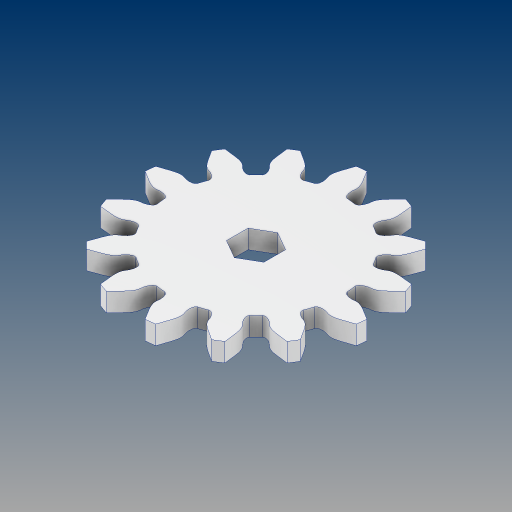
# Autodesk Inventor part: SHOT_1_016_5DP14TGear
Saved by Autodesk Inventor 2024.3 (Build 283343000, 343)
## iProperties
Created: 2024-08-09
Part Number: SHOT_1_016_5DP14TGear
Material: Aluminum 6061
Document SubType Name: Modeling
Designer: Kenji
Density: 2.7 g/cm^3
Appearance: Aluminum - Flat
Author: Kenji
Autodesk Inventor part; units mm, degrees
ref_plane "YZ Plane" through (0, 0, 0) normal (1, 0, 0) x (0, 1, 0)
ref_plane "XZ Plane" through (0, 0, 0) normal (0, 1, 0) x (-1, 0, 0)
ref_plane "XY Plane" through (0, 0, 0) normal (0, 0, 1) x (1, 0, 0)
sketch "Sketch3" plane through (0, 0, 0) normal (0, 1, 0) x (-1, 0, 0)
  circle A0 centre (0, 0) radius 40.64
  circle A1 centre (0, 0) radius 35.56 construction
  line L0 (0, 0) -> (0, -35.56) construction
  line L1 (0, 0) -> (11.4288, -31.4003) construction
  line L2 (11.4288, -31.4003) -> (0, -35.56) construction
  arc A2 (11.4288, -31.4003) -> (20.9412, -26.0395) centre (0, 0) ccw construction
  arc A3 (-0.498, -33.4118) -> (11.4288, -31.4003) centre (0, 0) ccw construction
  line L3 (20.9412, -26.0395) -> (2.9165, -40.5352) construction
  line L4 (0, -35.56) -> (-0.498, -33.4118) construction
  line L5 (26.4425, -30.8611) -> (-29.9661, -27.4526) construction
  line L6 (-0.498, -33.4118) -> (-1.7618, -29.1568) construction
  line L7 (15.9914, -37.3615) -> (-36.81, -17.2231) construction
  line L8 (-0.498, -33.4118) -> (-0.4624, -31.086) construction
  line L9 (-0.4624, -31.086) -> (-1.7618, -29.1568) construction
  line L10 (12.7503, -38.5881) -> (-38.1434, -14.0245) construction
  line L11 (-0.498, -33.4118) -> (-0.3808, -32.2504) construction
  line L12 (-0.3808, -32.2504) -> (-0.4624, -31.086) construction
  line L13 (20.121, -35.3094) -> (-34.6219, -21.2823) construction
  line L14 (-0.498, -33.4118) -> (-0.8403, -29.9384) construction
  line L15 (-0.8403, -29.9384) -> (-1.7618, -29.1568) construction
  line L16 (-0.4624, -31.086) -> (-0.8403, -29.9384) construction
  line L17 (0, 0) -> (-3.2705, -29.0263) construction
  circle A4 centre (0, 0) radius 29.21 construction
  spline S0 degree 4 poles (2.9165, -40.5352) (1.7773, -38.368) (-1.3084, -34.6409) (0.0656, -32.8612) (-0.5512, -30.4753) (-0.8986, -29.4269) (-1.7618, -29.1568) knots 0 0 0 0 0 0.524578 0.668441 1 1 1 1 1
  arc A5 (-3.2705, -29.0263) -> (-1.7618, -29.1568) centre (0, 0) ccw
  spline S1 degree 4 poles (-11.8633, -38.8699) (-10.2705, -37.0106) (-6.4328, -34.0635) (-7.3763, -32.0227) (-6.244, -29.8339) (-5.672, -28.889) (-4.7704, -28.8178) knots 0 0 0 0 0 0.524578 0.668441 1 1 1 1 1
  arc A6 (-4.7704, -28.8178) -> (-3.2705, -29.0263) centre (0, 0) ccw
  arc A7 (9.6475, -27.5708) -> (11.0634, -27.0338) centre (0, 0) ccw
  arc A8 (8.2056, -28.0338) -> (9.6475, -27.5708) centre (0, 0) ccw
  spline S2 degree 4 poles (6.1766, -40.1679) (6.8049, -37.8016) (8.9839, -33.4812) (7.2483, -32.0519) (7.3188, -29.5886) (7.4242, -28.4891) (8.2056, -28.0338) knots 0 0 0 0 0 0.524578 0.668441 1 1 1 1 1
  spline S3 degree 4 poles (20.2152, -35.2555) (18.2486, -33.7973) (13.8513, -31.778) (14.3171, -29.5785) (12.7261, -27.6965) (11.9582, -26.9026) (11.0634, -27.0338) knots 0 0 0 0 0 0.524578 0.668441 1 1 1 1 1
  arc A9 (20.6546, -20.6546) -> (21.6973, -19.5564) centre (0, 0) ccw
  arc A10 (19.5564, -21.6973) -> (20.6546, -20.6546) centre (0, 0) ccw
  spline S4 degree 4 poles (22.9931, -33.5101) (22.5325, -31.1055) (22.6211, -26.2676) (20.4373, -25.7329) (19.432, -23.4829) (19.0499, -22.4466) (19.5564, -21.6973) knots 0 0 0 0 0 0.524578 0.668441 1 1 1 1 1
  spline S5 degree 4 poles (33.5101, -22.9931) (31.1055, -22.5325) (26.2676, -22.6211) (25.7329, -20.4373) (23.4829, -19.432) (22.4466, -19.0499) (21.6973, -19.5564) knots 0 0 0 0 0 0.524578 0.668441 1 1 1 1 1
  arc A11 (27.5708, -9.6475) -> (28.0338, -8.2056) centre (0, 0) ccw
  arc A12 (27.0338, -11.0634) -> (27.5708, -9.6475) centre (0, 0) ccw
  spline S6 degree 4 poles (35.2555, -20.2152) (33.7973, -18.2486) (31.778, -13.8513) (29.5785, -14.3171) (27.6965, -12.7261) (26.9026, -11.9582) (27.0338, -11.0634) knots 0 0 0 0 0 0.524578 0.668441 1 1 1 1 1
  spline S7 degree 4 poles (40.1679, -6.1766) (37.8016, -6.8049) (33.4812, -8.9839) (32.0519, -7.2483) (29.5886, -7.3188) (28.4891, -7.4242) (28.0338, -8.2056) knots 0 0 0 0 0 0.524578 0.668441 1 1 1 1 1
  arc A13 (29.0263, 3.2705) -> (28.8178, 4.7704) centre (0, 0) ccw
  arc A14 (29.1568, 1.7618) -> (29.0263, 3.2705) centre (0, 0) ccw
  spline S8 degree 4 poles (40.5352, -2.9165) (38.368, -1.7773) (34.6409, 1.3084) (32.8612, -0.0656) (30.4753, 0.5512) (29.4269, 0.8986) (29.1568, 1.7618) knots 0 0 0 0 0 0.524578 0.668441 1 1 1 1 1
  spline S9 degree 4 poles (38.8699, 11.8633) (37.0106, 10.2705) (34.0635, 6.4328) (32.0227, 7.3763) (29.8339, 6.244) (28.889, 5.672) (28.8178, 4.7704) knots 0 0 0 0 0 0.524578 0.668441 1 1 1 1 1
  arc A15 (24.7328, 15.5407) -> (23.8942, 16.8016) centre (0, 0) ccw
  arc A16 (25.505, 14.238) -> (24.7328, 15.5407) centre (0, 0) ccw
  spline S10 degree 4 poles (37.7864, 14.9599) (35.3396, 15.046) (30.6427, 16.2089) (29.6354, 14.1988) (27.2182, 13.7194) (26.1228, 13.5775) (25.505, 14.238) knots 0 0 0 0 0 0.524578 0.668441 1 1 1 1 1
  spline S11 degree 4 poles (29.8733, 27.5535) (28.8892, 25.3117) (27.8991, 20.5753) (25.651, 20.54) (24.1703, 18.5701) (23.5671, 17.6448) (23.8942, 16.8016) knots 0 0 0 0 0 0.524578 0.668441 1 1 1 1 1
  arc A17 (15.5407, 24.7328) -> (14.238, 25.505) centre (0, 0) ccw
  arc A18 (16.8016, 23.8942) -> (15.5407, 24.7328) centre (0, 0) ccw
  spline S12 degree 4 poles (27.5535, 29.8733) (25.3117, 28.8892) (20.5753, 27.8991) (20.54, 25.651) (18.5701, 24.1703) (17.6448, 23.5671) (16.8016, 23.8942) knots 0 0 0 0 0 0.524578 0.668441 1 1 1 1 1
  spline S13 degree 4 poles (14.9599, 37.7864) (15.046, 35.3396) (16.2089, 30.6427) (14.1988, 29.6354) (13.7194, 27.2182) (13.5775, 26.1228) (14.238, 25.505) knots 0 0 0 0 0 0.524578 0.668441 1 1 1 1 1
  arc A19 (3.2705, 29.0263) -> (1.7618, 29.1568) centre (0, 0) ccw
  arc A20 (4.7704, 28.8178) -> (3.2705, 29.0263) centre (0, 0) ccw
  spline S14 degree 4 poles (11.8633, 38.8699) (10.2705, 37.0106) (6.4328, 34.0635) (7.3763, 32.0227) (6.244, 29.8339) (5.672, 28.889) (4.7704, 28.8178) knots 0 0 0 0 0 0.524578 0.668441 1 1 1 1 1
  spline S15 degree 4 poles (-2.9165, 40.5352) (-1.7773, 38.368) (1.3084, 34.6409) (-0.0656, 32.8612) (0.5512, 30.4753) (0.8986, 29.4269) (1.7618, 29.1568) knots 0 0 0 0 0 0.524578 0.668441 1 1 1 1 1
  arc A21 (-9.6475, 27.5708) -> (-11.0634, 27.0338) centre (0, 0) ccw
  arc A22 (-8.2056, 28.0338) -> (-9.6475, 27.5708) centre (0, 0) ccw
  spline S16 degree 4 poles (-6.1766, 40.1679) (-6.8049, 37.8016) (-8.9839, 33.4812) (-7.2483, 32.0519) (-7.3188, 29.5886) (-7.4242, 28.4891) (-8.2056, 28.0338) knots 0 0 0 0 0 0.524578 0.668441 1 1 1 1 1
  spline S17 degree 4 poles (-20.2152, 35.2555) (-18.2486, 33.7973) (-13.8513, 31.778) (-14.3171, 29.5785) (-12.7261, 27.6965) (-11.9582, 26.9026) (-11.0634, 27.0338) knots 0 0 0 0 0 0.524578 0.668441 1 1 1 1 1
  arc A23 (-20.6546, 20.6546) -> (-21.6973, 19.5564) centre (0, 0) ccw
  arc A24 (-19.5564, 21.6973) -> (-20.6546, 20.6546) centre (0, 0) ccw
  spline S18 degree 4 poles (-22.9931, 33.5101) (-22.5325, 31.1055) (-22.6211, 26.2676) (-20.4373, 25.7329) (-19.432, 23.4829) (-19.0499, 22.4466) (-19.5564, 21.6973) knots 0 0 0 0 0 0.524578 0.668441 1 1 1 1 1
  spline S19 degree 4 poles (-33.5101, 22.9931) (-31.1055, 22.5325) (-26.2676, 22.6211) (-25.7329, 20.4373) (-23.4829, 19.432) (-22.4466, 19.0499) (-21.6973, 19.5564) knots 0 0 0 0 0 0.524578 0.668441 1 1 1 1 1
  arc A25 (-27.5708, 9.6475) -> (-28.0338, 8.2056) centre (0, 0) ccw
  arc A26 (-27.0338, 11.0634) -> (-27.5708, 9.6475) centre (0, 0) ccw
  spline S20 degree 4 poles (-35.2555, 20.2152) (-33.7973, 18.2486) (-31.778, 13.8513) (-29.5785, 14.3171) (-27.6965, 12.7261) (-26.9026, 11.9582) (-27.0338, 11.0634) knots 0 0 0 0 0 0.524578 0.668441 1 1 1 1 1
  spline S21 degree 4 poles (-40.1679, 6.1766) (-37.8016, 6.8049) (-33.4812, 8.9839) (-32.0519, 7.2483) (-29.5886, 7.3188) (-28.4891, 7.4242) (-28.0338, 8.2056) knots 0 0 0 0 0 0.524578 0.668441 1 1 1 1 1
  arc A27 (-29.0263, -3.2705) -> (-28.8178, -4.7704) centre (0, 0) ccw
  arc A28 (-29.1568, -1.7618) -> (-29.0263, -3.2705) centre (0, 0) ccw
  spline S22 degree 4 poles (-40.5352, 2.9165) (-38.368, 1.7773) (-34.6409, -1.3084) (-32.8612, 0.0656) (-30.4753, -0.5512) (-29.4269, -0.8986) (-29.1568, -1.7618) knots 0 0 0 0 0 0.524578 0.668441 1 1 1 1 1
  spline S23 degree 4 poles (-38.8699, -11.8633) (-37.0106, -10.2705) (-34.0635, -6.4328) (-32.0227, -7.3763) (-29.8339, -6.244) (-28.889, -5.672) (-28.8178, -4.7704) knots 0 0 0 0 0 0.524578 0.668441 1 1 1 1 1
  arc A29 (-24.7328, -15.5407) -> (-23.8942, -16.8016) centre (0, 0) ccw
  arc A30 (-25.505, -14.238) -> (-24.7328, -15.5407) centre (0, 0) ccw
  spline S24 degree 4 poles (-37.7864, -14.9599) (-35.3396, -15.046) (-30.6427, -16.2089) (-29.6354, -14.1988) (-27.2182, -13.7194) (-26.1228, -13.5775) (-25.505, -14.238) knots 0 0 0 0 0 0.524578 0.668441 1 1 1 1 1
  spline S25 degree 4 poles (-29.8733, -27.5535) (-28.8892, -25.3117) (-27.8991, -20.5753) (-25.651, -20.54) (-24.1703, -18.5701) (-23.5671, -17.6448) (-23.8942, -16.8016) knots 0 0 0 0 0 0.524578 0.668441 1 1 1 1 1
  arc A31 (-15.5407, -24.7328) -> (-14.238, -25.505) centre (0, 0) ccw
  arc A32 (-16.8016, -23.8942) -> (-15.5407, -24.7328) centre (0, 0) ccw
  spline S26 degree 4 poles (-27.5535, -29.8733) (-25.3117, -28.8892) (-20.5753, -27.8991) (-20.54, -25.651) (-18.5701, -24.1703) (-17.6448, -23.5671) (-16.8016, -23.8942) knots 0 0 0 0 0 0.524578 0.668441 1 1 1 1 1
  spline S27 degree 4 poles (-14.9599, -37.7864) (-15.046, -35.3396) (-16.2089, -30.6427) (-14.1988, -29.6354) (-13.7194, -27.2182) (-13.5775, -26.1228) (-14.238, -25.505) knots 0 0 0 0 0 0.524578 0.668441 1 1 1 1 1
  circle A33 centre (0, 0) radius 40.64 construction
  point P0 (0, -35.56)
  point P1 (-6.4665, -30.4095)
  point P2 (-7.9128, -34.6684)
  point P3 (-6.9493, -32.6849)
  point P4 (-6.8051, -31.5266)
  point P5 (-5.8427, -29.3747)
  point P6 (7.9128, -34.6684)
  point P7 (7.9203, -32.4632)
  point P8 (7.5476, -31.3571)
  point P9 (7.3681, -30.2037)
  point P10 (7.4811, -29.0008)
  point P11 (15.4289, -32.0385)
  point P12 (14.0481, -30.319)
  point P13 (13.6499, -29.2218)
  point P14 (13.0711, -28.2082)
  point P15 (12.2327, -27.3381)
  point P16 (22.1713, -27.8019)
  point P17 (21.2213, -25.8119)
  point P18 (20.4055, -24.977)
  point P19 (19.7434, -24.0157)
  point P20 (19.3232, -22.8828)
  point P21 (27.8019, -22.1713)
  point P22 (25.8119, -21.2213)
  point P23 (24.977, -20.4055)
  point P24 (24.0157, -19.7434)
  point P25 (22.8828, -19.3232)
  point P26 (32.0385, -15.4289)
  point P27 (30.319, -14.0481)
  point P28 (29.2218, -13.6499)
  point P29 (28.2082, -13.0711)
  point P30 (27.3381, -12.2327)
  point P31 (34.6684, -7.9128)
  point P32 (32.4632, -7.9203)
  point P33 (31.3571, -7.5476)
  point P34 (30.2037, -7.3681)
  point P35 (29.0008, -7.4811)
  point P36 (35.56, 0)
  point P37 (33.4118, 0.498)
  point P38 (32.2504, 0.3808)
  point P39 (31.086, 0.4624)
  point P40 (29.9384, 0.8403)
  point P41 (34.6684, 7.9128)
  point P42 (32.6849, 6.9493)
  point P43 (31.5266, 6.8051)
  point P44 (30.4095, 6.4665)
  point P45 (29.3747, 5.8427)
  point P46 (32.0385, 15.4289)
  point P47 (29.8869, 14.9455)
  point P48 (28.8914, 14.336)
  point P49 (27.8069, 13.9044)
  point P50 (26.6089, 13.7469)
  point P51 (27.8019, 22.1713)
  point P52 (26.4329, 20.4425)
  point P53 (25.4518, 19.8101)
  point P54 (24.5924, 19.0203)
  point P55 (23.9307, 18.0093)
  point P56 (22.1713, 27.8019)
  point P57 (20.4425, 26.4329)
  point P58 (19.8101, 25.4518)
  point P59 (19.0203, 24.5924)
  point P60 (18.0093, 23.9307)
  point P61 (15.4289, 32.0385)
  point P62 (14.9455, 29.8869)
  point P63 (14.336, 28.8914)
  point P64 (13.9044, 27.8069)
  point P65 (13.7469, 26.6089)
  point P66 (7.9128, 34.6684)
  point P67 (6.9493, 32.6849)
  point P68 (6.8051, 31.5266)
  point P69 (6.4665, 30.4095)
  point P70 (5.8427, 29.3747)
  point P71 (0, 35.56)
  point P72 (0.498, 33.4118)
  point P73 (0.3808, 32.2504)
  point P74 (0.4624, 31.086)
  point P75 (0.8403, 29.9384)
  point P76 (-7.9128, 34.6684)
  point P77 (-7.9203, 32.4632)
  point P78 (-7.5476, 31.3571)
  point P79 (-7.3681, 30.2037)
  point P80 (-7.4811, 29.0008)
  point P81 (-15.4289, 32.0385)
  point P82 (-14.0481, 30.319)
  point P83 (-13.6499, 29.2218)
  point P84 (-13.0711, 28.2082)
  point P85 (-12.2327, 27.3381)
  point P86 (-22.1713, 27.8019)
  point P87 (-21.2213, 25.8119)
  point P88 (-20.4055, 24.977)
  point P89 (-19.7434, 24.0157)
  point P90 (-19.3232, 22.8828)
  point P91 (-27.8019, 22.1713)
  point P92 (-25.8119, 21.2213)
  point P93 (-24.977, 20.4055)
  point P94 (-24.0157, 19.7434)
  point P95 (-22.8828, 19.3232)
  point P96 (-32.0385, 15.4289)
  point P97 (-30.319, 14.0481)
  point P98 (-29.2218, 13.6499)
  point P99 (-28.2082, 13.0711)
  point P100 (-27.3381, 12.2327)
  point P101 (-34.6684, 7.9128)
  point P102 (-32.4632, 7.9203)
  point P103 (-31.3571, 7.5476)
  point P104 (-30.2037, 7.3681)
  point P105 (-29.0008, 7.4811)
  point P106 (-35.56, 0)
  point P107 (-33.4118, -0.498)
  point P108 (-32.2504, -0.3808)
  point P109 (-31.086, -0.4624)
  point P110 (-29.9384, -0.8403)
  point P111 (-34.6684, -7.9128)
  point P112 (-32.6849, -6.9493)
  point P113 (-31.5266, -6.8051)
  point P114 (-30.4095, -6.4665)
  point P115 (-29.3747, -5.8427)
  point P116 (-32.0385, -15.4289)
  point P117 (-29.8869, -14.9455)
  point P118 (-28.8914, -14.336)
  point P119 (-27.8069, -13.9044)
  point P120 (-26.6089, -13.7469)
  point P121 (-27.8019, -22.1713)
  point P122 (-26.4329, -20.4425)
  point P123 (-25.4518, -19.8101)
  point P124 (-24.5924, -19.0203)
  point P125 (-23.9307, -18.0093)
  point P126 (-22.1713, -27.8019)
  point P127 (-20.4425, -26.4329)
  point P128 (-19.8101, -25.4518)
  point P129 (-19.0203, -24.5924)
  point P130 (-18.0093, -23.9307)
  point P131 (-15.4289, -32.0385)
  point P132 (-14.9455, -29.8869)
  point P133 (-14.336, -28.8914)
  point P134 (-13.9044, -27.8069)
  point P135 (-13.7469, -26.6089)
  point P136 (2.9165, -40.5352)
  point P137 (6.1766, -40.1679)
  point P138 (20.2152, -35.2555)
  point P139 (22.9931, -33.5101)
  point P140 (33.5101, -22.9931)
  point P141 (35.2555, -20.2152)
  point P142 (40.1679, -6.1766)
  point P143 (40.5352, -2.9165)
  point P144 (38.8699, 11.8633)
  point P145 (37.7864, 14.9599)
  point P146 (29.8733, 27.5535)
  point P147 (27.5535, 29.8733)
  point P148 (14.9599, 37.7864)
  point P149 (11.8633, 38.8699)
  point P150 (-2.9165, 40.5352)
  point P151 (-6.1766, 40.1679)
  point P152 (-20.2152, 35.2555)
  point P153 (-22.9931, 33.5101)
  point P154 (-33.5101, 22.9931)
  point P155 (-35.2555, 20.2152)
  point P156 (-40.1679, 6.1766)
  point P157 (-40.5352, 2.9165)
  point P158 (-38.8699, -11.8633)
  point P159 (-37.7864, -14.9599)
  point P160 (-29.8733, -27.5535)
  point P161 (-27.5535, -29.8733)
  point P162 (-14.9599, -37.7864)
  point P163 (-11.8633, -38.8699)
  dimension "d58" = 81.28
  dimension "d59" = 71.12
  dimension "d60" = 20
  dimension "d61" = 12.1622
  dimension "d62" = 12.1622
  dimension "d63" = 23.1304
  dimension "d64" = 10.9682
  dimension "d65" = 29.21
  dimension "d66" = 70
  dimension "d67" = 29.21
  dimension "d68" = 70
  dimension "d69" = 29.21
  dimension "d70" = 70
  dimension "d71" = 29.21
  dimension "d72" = 70
  dimension "d73" = 6.429
  dimension "d77" = 360
  constraints: 60 point on circle, 36 end point, 30 centre point, 11 coincident, 7 symmetric about line, 3 equal length, 3 point on line, 1 midpoint, 1 perpendicular, 1 tangent, 1 vertical, 1 vertical alignment, 501 other
  measures "d60" angle of L0 L1
  measures "d61" distance of L1.end L0.end
  measures "d63" distance of L3.start L3.end
  measures "d65" distance from line of point (0, 0) L5
  measures "d66" angle of L5 L6
  measures "d67" distance from line of point (0, 0) L7
  measures "d68" angle of L7 L8
  measures "d69" distance from line of point (0, 0) L10
  measures "d70" angle of L10 L11
  measures "d71" distance from line of point (0, 0) L13
  measures "d72" angle of L13 L14
  measures "d73" angle of L0 L17
extrude "Extrusion3" add sketch "Sketch3" along normal blind 6.35 contours S9 A13 A14 S8 A0 S7 A11 A12 S6 S5 A9 A10 S4 S3 A7 A8 S2 S0 A5 A6 S1 S27 A31 A32 S26 S25 A29 A30 S24 S23 A27 A28 S22 S21 A25 A26 S20 S19 A23 A24 S18 S17 A21 A22 S16 S15 A19 A20 S14 S13 A17 A18 S12 S11 A15 A16 S10
sketch "Sketch4" plane through (0, 6.35, 0) normal (0, 1, 0) x (1, 0, 0)
  line L0 (-6.35, 3.6662) -> (0, 7.3323)
  line L1 (0, 7.3323) -> (6.35, 3.6662)
  line L2 (6.35, 3.6662) -> (6.35, -3.6662)
  line L3 (6.35, -3.6662) -> (0, -7.3323)
  line L4 (0, -7.3323) -> (-6.35, -3.6662)
  line L5 (-6.35, -3.6662) -> (-6.35, 3.6662)
  point P0 (0, 0)
  point P1 (0, 0)
  dimension "d81" = 12.7
  constraints: 12 end point, 1 coincident, 13 other
  measures "d81" distance between parallel lines of L2 L5
extrude "Extrusion4" cut sketch "Sketch4" against normal blind 6.35
body "Solid2"
